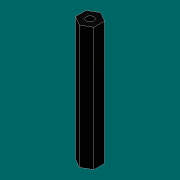
# Autodesk Inventor part: AMP-340E
Saved by Autodesk Inventor 2016 (Build 200138000, 138)
## iProperties
Created: 2016-08-26
Part Number: AMP-340E
Material: PPS プラスチック
Document SubType Name: Modeling
Designer: hiro
Density: 1.637 g/cm^3
Appearance: 滑らか - 黒
Mass: 1.74524 g
Surface Area: 11.8628 cm^2
Volume: 1.06612 cm^3
Author: hiro
Autodesk Inventor part; units mm, degrees
ref_plane "YZ Plane" through (0, 0, 0) normal (1, 0, 0) x (0, 1, 0)
ref_plane "XZ Plane" through (0, 0, 0) normal (0, 1, 0) x (-1, 0, 0)
ref_plane "XY Plane" through (0, 0, 0) normal (0, 0, 1) x (1, 0, 0)
sketch "スケッチ1" plane through (0, 0, 0) normal (0, 0, 1) x (1, 0, 0)
  line L0 (3, 1.7321) -> (3, -1.7321)
  line L1 (3, -1.7321) -> (0, -3.4641)
  line L2 (0, -3.4641) -> (-3, -1.7321)
  line L3 (-3, -1.7321) -> (-3, 1.7321)
  line L4 (-3, 1.7321) -> (0, 3.4641)
  line L5 (0, 3.4641) -> (3, 1.7321)
  circle A0 centre (0, 0) radius 1.2
  dimension "d0" = 2.4
  dimension "d1" = 6
  constraints: 12 end point, 2 coincident, 1 centre point, 1 vertical, 13 other
  measures "d0" diameter of A0
  measures "d1" distance between parallel lines of L0 L3
extrude "押し出し1" add sketch "スケッチ1" along normal blind 40
